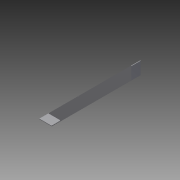
# Autodesk Inventor part: electronics board support outside
Saved by Autodesk Inventor 2012 (Build 160160000, 160)
## iProperties
Created: 2013-10-05
Part Number: electronics board support outside
Material: Default
Document SubType Name: Modeling
Designer: Bryce
Density: 1 g/cm^3
Author: Bryce
Autodesk Inventor part; units mm, degrees
ref_plane "YZ Plane" through (0, 0, 0) normal (1, 0, 0) x (0, 1, 0)
ref_plane "XZ Plane" through (0, 0, 0) normal (0, 1, 0) x (-1, 0, 0)
ref_plane "XY Plane" through (0, 0, 0) normal (0, 0, 1) x (1, 0, 0)
sketch "Sketch1" plane through (0, 0, 0) normal (0, 0, 1) x (1, 0, 0)
  line L0 (0, 0) -> (34.3335, 0)
  line L1 (33.676, 1.5875) -> (0, 1.5875)
  line L2 (0, 1.5875) -> (0, 0)
  line L3 (34.3335, 0) -> (254, 219.6665)
  line L4 (1.1112, 2.6987) -> (251.3012, 252.8888)
  line L5 (33.676, 1.5875) -> (252.4125, 220.324)
  line L6 (1.1112, 2.6987) -> (32.0885, 2.6988)
  arc A0 (32.0885, 1.5875) -> (32.0885, 2.6988) centre (32.0885, 2.1431) ccw
  line L7 (252.4125, 220.324) -> (252.4125, 254)
  line L8 (252.4125, 254) -> (254, 254)
  line L9 (254, 254) -> (254, 219.6665)
  line L10 (251.3012, 252.8888) -> (251.3012, 221.9115)
  arc A1 (251.3012, 221.9115) -> (252.4125, 221.9115) centre (251.8569, 221.9115) ccw
  dimension "d0" = 25.4
  dimension "d1" = 135
  dimension "d2" = 1.5875
  dimension "d3" = 1.5875
  dimension "d4" = 1.1113
  dimension "d5" = 1.5875
  dimension "d6" = 1.5875
  dimension "d7" = 254
  dimension "d9" = 1.1113
  dimension "d10" = 1.5875
  constraints: 22 end point, 5 parallel, 4 point on circle, 4 point on line, 4 tangent, 3 perpendicular, 2 centre point, 1 horizontal
  measures "d0" distance between parallel lines of L3 L4
  measures "d1" angle of L0 L3
  measures "d2" distance of L1.end L0.start
  measures "d3" distance between parallel lines of L3 L5
  measures "d4" distance between parallel lines of L1 L6
  measures "d5" horizontal distance of L1.start A0.centre
  measures "d6" distance of L7.end L8.end
  measures "d7" distance between parallel lines of L2 L9
  measures "d9" distance between parallel lines of L7 L10
  measures "d10" vertical distance of L5.end A1.centre
extrude "Extrusion1" add sketch "Sketch1" along normal blind 1.5875 contours A0 L6 L4 L10 A1 L7 L5 L1
extrude "Extrusion2" add sketch "Sketch1" along normal blind 25.4 contours L2 L1 L5 L7 L8 L9 L3 L0
equation "\"d3\" = d2"
equation "\"d4\" = 0.7 * d2"
equation "\"d5\" = d2"
equation "\"d6\" = d2"
equation "\"d9\" = d4"
equation "\"d10\" = d6"
body "Solid1"
